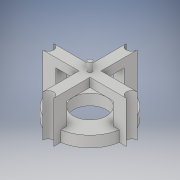
# Autodesk Inventor part: CheckValveValve1.0
Saved by Autodesk Inventor 2019 (Build 230136000, 136)
## iProperties
Created: 2019-04-04
Part Number: CheckValveValve1.0
Material: Generic
Document SubType Name: Modeling
Designer: Kepler
Density: 1 g/cm^3
Appearance: Default
Author: Kepler
Autodesk Inventor part; units mm, degrees
ref_plane "YZ Plane" through (0, 0, 0) normal (1, 0, 0) x (0, 1, 0)
ref_plane "XZ Plane" through (0, 0, 0) normal (0, 1, 0) x (-1, 0, 0)
ref_plane "XY Plane" through (0, 0, 0) normal (0, 0, 1) x (1, 0, 0)
sketch "Sketch9" plane through (0, 0, 0) normal (0, 1, 0) x (-1, 0, 0)
  arc A0 (19, 2.5) -> (19, -2.5) centre (19, 0) ccw
  arc A1 (2.5, -19) -> (-2.5, -19) centre (0, -19) ccw
  arc A2 (-19, -2.5) -> (-19, 2.5) centre (-19, 0) ccw
  arc A3 (-2.5, 19) -> (2.5, 19) centre (0, 19) ccw
  line L0 (-2.5, 19) -> (-2.5, 15.8035)
  line L1 (2.5, 19) -> (2.5, 15.8035)
  line L2 (19, 2.5) -> (15.8035, 2.5)
  line L3 (19, -2.5) -> (15.8035, -2.5)
  line L4 (-19, -2.5) -> (-15.8035, -2.5)
  line L5 (-19, 2.5) -> (-15.8035, 2.5)
  line L6 (-2.5, -19) -> (-2.5, -15.8035)
  line L7 (2.5, -19) -> (2.5, -15.8035)
  arc A4 (-2.5, 15.8035) -> (-15.8035, 2.5) centre (0, 0) ccw
  arc A5 (15.8035, 2.5) -> (2.5, 15.8035) centre (0, 0) ccw
  arc A6 (-15.8035, -2.5) -> (-2.5, -15.8035) centre (0, 0) ccw
  arc A7 (2.5, -15.8035) -> (15.8035, -2.5) centre (0, 0) ccw
  circle A8 centre (0, 0) radius 7.5
  dimension "d49" = 2.5
  dimension "d50" = 2.5
  dimension "d51" = 2.5
  dimension "d52" = 2.5
  dimension "d53" = 16
  dimension "d54" = 16
  dimension "d55" = 16
  dimension "d56" = 16
  dimension "d59" = 15
  constraints: 17 point on circle, 16 end point, 9 centre point, 4 point on line, 2 coincident, 2 tangent, 1 parallel, 1 perpendicular, 1 vertical
  measures "d49" radius of A0
  measures "d50" radius of A1
  measures "d51" radius of A2
  measures "d52" radius of A3
  measures "d53" radius of A7
  measures "d54" radius of A5
  measures "d55" radius of A4
  measures "d56" radius of A6
  measures "d59" diameter of A8
extrude "Extrusion10" add sketch "Sketch9" along normal blind 5
sketch "Sketch10" plane through (0, 0, 0) normal (0, -1, 0) x (1, 0, 0)
  circle A0 centre (0, 0) radius 8.5
  circle A1 centre (0, 0) radius 15
  dimension "d62" = 17
  dimension "d63" = 30
  constraints: 2 centre point, 2 coincident
  measures "d62" diameter of A0
  measures "d63" diameter of A1
extrude "Extrusion11" cut sketch "Sketch10" against normal blind 1
sketch "Sketch11" plane through (0, 5, 0) normal (0, 1, 0) x (1, 0, 0)
  arc A0 (19, 2.5) -> (19, -2.5) centre (19, 0) ccw projected
  arc A1 (19, 2.5) -> (19, -2.5) centre (19, 0) ccw
  arc A2 (-2.5, 19) -> (2.5, 19) centre (0, 19) ccw projected
  arc A3 (-2.5, 19) -> (2.5, 19) centre (0, 19) ccw
  arc A4 (-19, -2.5) -> (-19, 2.5) centre (-19, 0) ccw projected
  arc A5 (-19, -2.5) -> (-19, 2.5) centre (-19, 0) ccw
  line L0 (2.5, -15.8035) -> (2.5, -19) projected
  arc A6 (2.5, -19) -> (-2.5, -19) centre (0, -19) ccw
  line L1 (2.5, -19) -> (2.5, -13)
  line L2 (2.5, -13) -> (-2.5, -13)
  line L3 (-2.5, -19) -> (-2.5, -15.8035) projected
  line L4 (-2.5, -13) -> (-2.5, -19)
  line L5 (-19, -2.5) -> (-13, -2.5)
  line L6 (-13, -2.5) -> (-13, 2.5)
  line L7 (-13, 2.5) -> (-19, 2.5)
  line L8 (-2.5, 19) -> (-2.5, 13)
  line L9 (-2.5, 13) -> (2.5, 13)
  line L10 (2.5, 13) -> (2.5, 19)
  line L11 (15.8035, 2.5) -> (19, 2.5) projected
  line L12 (19, 2.5) -> (13, 2.5)
  line L13 (13, 2.5) -> (13, -2.5)
  line L14 (13, -2.5) -> (19, -2.5)
  point P0 (0, 0)
  constraints: 24 end point, 10 point on circle, 8 perpendicular, 7 tangent, 4 centre point, 2 point on line, 2 vertical, 1 horizontal
extrude "Extrusion12" add sketch "Sketch11" along normal blind 10
sketch "Sketch12" plane through (0, 15, 0) normal (0, 1, 0) x (1, 0, 0)
  line L0 (19, -2.5) -> (15.8035, -2.5) projected
  line L1 (2.5, -2.5) -> (2.5, -19)
  line L2 (2.5, -13) -> (2.5, -15.8035) projected
  arc A0 (2.5, -19) -> (-2.5, -19) centre (0, -19) ccw
  arc A1 (-19, -2.5) -> (-19, 2.5) centre (-19, 0) ccw
  arc A2 (-2.5, 19) -> (2.5, 19) centre (0, 19) ccw projected
  arc A3 (-2.5, 19) -> (2.5, 19) centre (0, 19) ccw
  arc A4 (19, 2.5) -> (19, -2.5) centre (19, 0) ccw
  arc A5 (2.5, -19) -> (-2.5, -19) centre (0, -19) ccw projected
  line L3 (-2.5, -19) -> (-2.5, -2.5)
  line L4 (-2.5, -2.5) -> (-19, -2.5)
  line L5 (-19, 2.5) -> (-2.5, 2.5)
  line L6 (-2.5, 15.8035) -> (-2.5, 19) projected
  line L7 (-2.5, 2.5) -> (-2.5, 19)
  line L8 (2.5, 19) -> (2.5, 2.5)
  line L9 (15.8035, 2.5) -> (19, 2.5) projected
  line L10 (2.5, 2.5) -> (19, 2.5)
  line L11 (2.5, -2.5) -> (2.5, 2.5)
  line L12 (2.5, 2.5) -> (-2.5, 2.5)
  line L13 (-2.5, -2.5) -> (-2.5, 2.5)
  line L14 (-2.5, -2.5) -> (2.5, -2.5)
  arc A6 (19, 2.5) -> (19, -2.5) centre (19, 0) ccw projected
  line L15 (19, -2.5) -> (2.5, -2.5)
  point P0 (0, 0)
  dimension "d68" = 5
  dimension "d70" = 0
  dimension "d71" = 21.5
  constraints: 24 end point, 11 tangent, 8 point on circle, 4 centre point, 3 perpendicular, 3 vertical, 2 collinear, 1 parallel, 1 point on line
  measures "d68" distance between parallel lines of L5 L0
  measures "d70" distance from line of A4.end L0
  measures "d71" distance from line of L5.start L2
extrude "Extrusion13" add sketch "Sketch12" along normal blind 4
sketch "Sketch13" plane through (0, 19, 0) normal (0, 1, 0) x (1, 0, 0)
  circle A0 centre (0, 0) radius 1
  dimension "d74" = 2
  constraints: 1 centre point, 1 coincident
  measures "d74" diameter of A0
extrude "Extrusion14" add sketch "Sketch13" along normal blind 4
equation "\"d54\" = d53"
equation "\"d55\" = d53"
equation "\"d56\" = d53"
body "Solid4"
